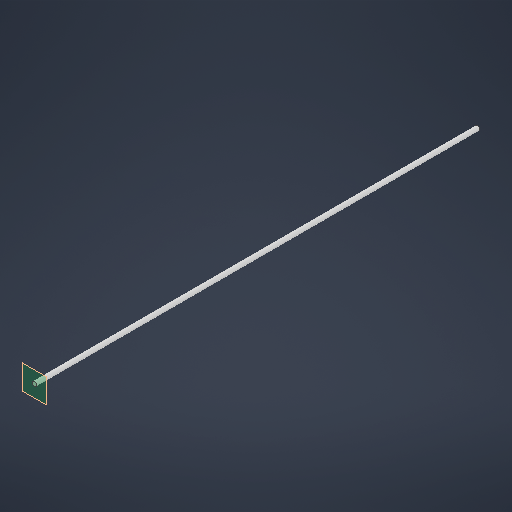
# Autodesk Inventor part: back_wheel_stick
Saved by Autodesk Inventor 2026.3 (Build 303398000, 398)
## iProperties
Created: 2026-08-06
Part Number: back_wheel_stick
Material: 일반
Document SubType Name: Modeling
Designer: hojin
Density: 1 g/cm^3
Appearance: 기본값
Author: hojin
Autodesk Inventor part; units mm, degrees
ref_plane "YZ Plane" through (0, 0, 0) normal (1, 0, 0) x (0, 1, 0)
ref_plane "XZ Plane" through (0, 0, 0) normal (0, 1, 0) x (-1, 0, 0)
ref_plane "XY Plane" through (0, 0, 0) normal (0, 0, 1) x (1, 0, 0)
sketch "스케치1" plane through (0, 0, 0) normal (1, 0, 0) x (0, 1, 0)
  line L0 (0, 200) -> (0, -200)
  point P0 (0, 0)
  point P1 (0, 0)
  dimension "d3" = 400
  constraints: 2 end point, 1 coincident, 1 midpoint, 1 vertical
  measures "d3" distance of L0.start L0.end
ref_plane "작업 평면1" through (0, 0, 200) normal (0, 0, -1) x (-1, 0, 0)
sketch "스케치2" plane through (0, 0, 200) normal (0, 0, -1) x (-1, 0, 0)
  circle A0 centre (0, 0) radius 2
  point P0 (0, 0)
  dimension "d0" = 4
  constraints: 1 centre point, 1 coincident
  measures "d0" diameter of A0
sweep "스윕1" add profiles "스케치2" path "스케치1"
